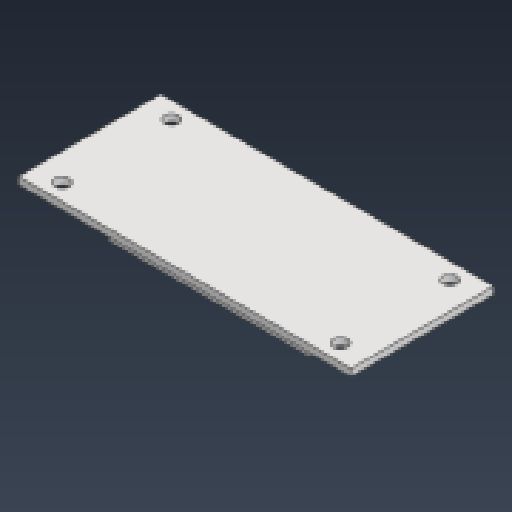
# Autodesk Inventor part: my_own_pcb
Saved by Autodesk Inventor 2023 (Build 270158000, 158)
## iProperties
Created: 2026-01-23
Part Number: my_own_pcb
Material: Generic
Document SubType Name: Modeling
Designer: szymo
Density: 1 g/cm^3
Appearance: Default
Author: szymo
Autodesk Inventor part; units mm, degrees
ref_plane "YZ Plane" through (0, 0, 0) normal (1, 0, 0) x (0, 1, 0)
ref_plane "XZ Plane" through (0, 0, 0) normal (0, 1, 0) x (-1, 0, 0)
ref_plane "XY Plane" through (0, 0, 0) normal (0, 0, 1) x (1, 0, 0)
sketch "Sketch1" plane through (0, 0, 0) normal (0, 1, 0) x (-1, 0, 0)
  line L0 (0, 0) -> (-70, 0)
  line L1 (-70, 0) -> (-70, -30)
  line L2 (-70, -30) -> (0, -30)
  line L3 (0, -30) -> (0, 0)
  circle A0 centre (-5.75, -3.5) radius 1.5
  circle A1 centre (-5.75, -26.5) radius 1.5
  circle A2 centre (-64.25, -3.5) radius 1.5
  circle A3 centre (-64.25, -26.5) radius 1.5
  line L4 (-5.75, -3.5) -> (-5.75, -26.5) construction
  line L5 (-5.75, -26.5) -> (-64.25, -26.5) construction
  line L6 (-64.25, -26.5) -> (-64.25, -3.5) construction
  line L7 (-64.25, -3.5) -> (-5.75, -3.5) construction
  dimension "d0" = 70
  dimension "d1" = 30
  dimension "d2" = 3
  dimension "d3" = 3
  dimension "d4" = 3
  dimension "d5" = 3
  dimension "d6" = 55.5
  dimension "d8" = 20
  dimension "d10" = 4.25
  dimension "d11" = 4.25
  dimension "d12" = 3.5
  dimension "d13" = 3.5
  constraints: 16 end point, 4 centre point, 3 horizontal, 3 parallel, 1 perpendicular, 1 vertical
  measures "d0" distance of L2.end L1.end
  measures "d1" distance of L1.end L0.end
  measures "d2" diameter of A0
  measures "d3" diameter of A1
  measures "d4" diameter of A2
  measures "d5" diameter of A3
  measures "d10" distance edge to line of A0 L3
  measures "d11" distance edge to line of A2 L1
  measures "d12" distance from line of L0 L4.start
  measures "d13" distance from line of L2 L4.end
extrude "Extrusion1" add sketch "Sketch1" along normal blind 1.5
sketch "Sketch2" plane through (0, 0, 0) normal (0, -1, 0) x (1, 0, 0)
  line L0 (12.3126, -6.7897) -> (54.4692, -6.7897)
  line L1 (54.4692, -6.7897) -> (54.4692, -21.3823)
  line L2 (54.4692, -21.3823) -> (12.3126, -21.3823)
  line L3 (12.3126, -21.3823) -> (12.3126, -6.7897)
  point P0 (0, 0)
  constraints: 8 end point, 2 parallel, 1 horizontal, 1 perpendicular
extrude "Extrusion2" add sketch "Sketch2" along normal blind 7.5
equation "\"d10\" = d11"
equation "\"d12\" = d13"
body "Solid1"
